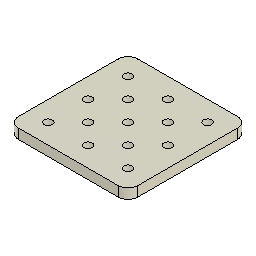
DrillingTool v1 (Autodesk Fusion 360 design; units mm, degrees)
Autodesk Fusion 360 part; units mm, degrees
note: some values were not read from the file. Set by a fixed rule: which sketch regions a step uses.
sketch "Sketch1" plane through (0, 0, 0) normal (0, 0, 1) x (1, 0, 0) in component "inside"
  line L0 (5, 0) -> (55, 0)
  line L1 (60, 5) -> (60, 55)
  line L2 (55, 60) -> (5, 60)
  line L3 (0, 55) -> (0, 5)
  circle A0 centre (10, 10) radius 2.05
  circle A1 centre (30, 10) radius 2.05
  circle A2 centre (10, 30) radius 2.05
  circle A3 centre (30, 30) radius 2.05
  circle A4 centre (50, 10) radius 2.05
  circle A5 centre (50, 30) radius 2.05
  circle A6 centre (20, 40) radius 2.05
  circle A7 centre (40, 40) radius 2.05
  circle A8 centre (10, 50) radius 2.05
  circle A9 centre (30, 50) radius 2.05
  circle A10 centre (50, 50) radius 2.05
  arc A11 (5, 60) -> (0, 55) centre (5, 55) ccw
  arc A12 (60, 55) -> (55, 60) centre (55, 55) ccw
  arc A13 (55, 0) -> (60, 5) centre (55, 5) ccw
  arc A14 (0, 5) -> (5, 0) centre (5, 5) ccw
  circle A15 centre (10, 20) radius 2.05
  circle A16 centre (30, 20) radius 2.05
  circle A17 centre (50, 20) radius 2.05
  circle A18 centre (10, 40) radius 2.05
  circle A19 centre (30, 40) radius 2.05
  circle A20 centre (50, 40) radius 2.05
  circle A21 centre (20, 50) radius 2.05
  circle A22 centre (40, 50) radius 2.05
  circle A23 centre (20, 10) radius 2.05
  circle A24 centre (40, 10) radius 2.05
  circle A25 centre (20, 20) radius 2.05
  circle A26 centre (40, 20) radius 2.05
  circle A27 centre (20, 30) radius 2.05
  circle A28 centre (40, 30) radius 2.05
  dimension "d6" = 60
  dimension "d7" = 60
  dimension "d9" = 4.1
  dimension "d10" = 10
  dimension "d11" = 10
  dimension "d14" = 10
  dimension "d15" = 10
  dimension "d17" = 5
  dimension "d18" = 5
  dimension "d19" = 5
  dimension "d20" = 5
  measures "d9" diameter of A0
  measures "d10" distance of origin
  measures "d11" distance of origin
  measures "d17" radius of A11
  measures "d18" radius of A12
  measures "d19" radius of A13
  measures "d20" radius of A14
extrude "Extrude1" add sketch "Sketch1" along normal blind 5 contours L0 L1 L2 L3 A11 A12 A13 A14 | A15 | A16 | A17 | A18 | A19 | A20 | A21 | A22 | A23 | A24 | A27 | A28 makes body 1 in component "inside"
sketch "Sketch1 (2)" plane through (0, 0, 0) normal (0, 0, 1) x (1, 0, 0) in component "inoutside"
  line L0 (0, -7.5) -> (60, -7.5)
  line L1 (60, -7.5) -> (60, 7.5)
  line L2 (60, 7.5) -> (0, 7.5)
  line L3 (0, 7.5) -> (0, -7.5)
  dimension "d23" = 15
  dimension "d24" = 60
sketch "Sketch2" plane through (0, 0, 0) normal (0, 1, 0) x (1, 0, 0) in component "inoutside"
  line L0 (0, 0) -> (60, 0)
  line L1 (60, 0) -> (60, -55)
  line L2 (55, -60) -> (5, -60)
  line L3 (0, -55) -> (0, 0)
  circle A0 centre (10, -10) radius 2.05
  circle A1 centre (20, -10) radius 2.05
  circle A2 centre (30, -10) radius 2.05
  circle A3 centre (40, -10) radius 2.05
  circle A4 centre (50, -10) radius 2.05
  circle A5 centre (10, -20) radius 2.05
  circle A6 centre (20, -20) radius 2.05
  circle A7 centre (30, -20) radius 2.05
  circle A8 centre (40, -20) radius 2.05
  circle A9 centre (50, -20) radius 2.05
  circle A10 centre (10, -30) radius 2.05
  circle A11 centre (20, -30) radius 2.05
  circle A12 centre (30, -30) radius 2.05
  circle A13 centre (40, -30) radius 2.05
  circle A14 centre (50, -30) radius 2.05
  circle A15 centre (10, -40) radius 2.05
  circle A16 centre (20, -40) radius 2.05
  circle A17 centre (30, -40) radius 2.05
  circle A18 centre (40, -40) radius 2.05
  circle A19 centre (50, -40) radius 2.05
  circle A20 centre (10, -50) radius 2.05
  circle A21 centre (20, -50) radius 2.05
  circle A22 centre (30, -50) radius 2.05
  circle A23 centre (40, -50) radius 2.05
  circle A24 centre (50, -50) radius 2.05
  arc A25 (0, -55) -> (5, -60) centre (5, -55) ccw
  arc A26 (55, -60) -> (60, -55) centre (55, -55) ccw
  dimension "d25" = 60
  dimension "d26" = 60
  dimension "d27" = 4.1
  dimension "d28" = 10
  dimension "d29" = 10
  dimension "d32" = 10
  dimension "d34" = 5
  dimension "d35" = 5
  measures "d27" diameter of A0
  measures "d28" distance of L0.start
  measures "d29" distance of L0.start
  measures "d34" radius of A25
  measures "d35" radius of A26
extrude "Extrude1'" add sketch "Sketch2" along normal mid plane 5 separate body contours L0 L1 L2 L3 A25 A26 | A1 | A3 | A5 | A7 | A9 | A11 | A13 | A15 | A17 | A19 | A21 | A23 makes body 2 in component "inoutside"
extrude "Extrude2" add sketch "Sketch1 (2)" against normal blind 5 bodies 2 in component "inoutside"
sketch "Sketch1 (3)" plane through (0, 0, 0) normal (0, 0, 1) x (1, 0, 0) in component "outside"
  line L0 (0, -7.5) -> (60, -7.5)
  line L1 (60, -7.5) -> (60, 7.5)
  line L2 (60, 7.5) -> (0, 7.5)
  line L3 (0, 7.5) -> (0, -7.5)
  line L4 (0, -7.5) -> (-5, -7.5)
  line L5 (-5, -7.5) -> (-5, 7.5)
  line L6 (-5, 7.5) -> (0, 7.5)
  line L7 (0, 7.5) -> (0, -7.5)
  dimension "d23_1" = 15
  dimension "d24_1" = 60
  dimension "d40" = 5
sketch "Sketch2 (2)" plane through (0, 0, 0) normal (0, 1, 0) x (1, 0, 0) in component "outside"
  line L0 (0, 0) -> (60, 0)
  line L1 (60, 0) -> (60, -55)
  line L2 (55, -60) -> (0, -60)
  line L3 (0, -60) -> (0, 0)
  circle A0 centre (10, -10) radius 2.05
  circle A1 centre (20, -10) radius 2.05
  circle A2 centre (30, -10) radius 2.05
  circle A3 centre (40, -10) radius 2.05
  circle A4 centre (50, -10) radius 2.05
  circle A5 centre (10, -20) radius 2.05
  circle A6 centre (20, -20) radius 2.05
  circle A7 centre (30, -20) radius 2.05
  circle A8 centre (40, -20) radius 2.05
  circle A9 centre (50, -20) radius 2.05
  circle A10 centre (10, -30) radius 2.05
  circle A11 centre (20, -30) radius 2.05
  circle A12 centre (30, -30) radius 2.05
  circle A13 centre (40, -30) radius 2.05
  circle A14 centre (50, -30) radius 2.05
  circle A15 centre (10, -40) radius 2.05
  circle A16 centre (20, -40) radius 2.05
  circle A17 centre (30, -40) radius 2.05
  circle A18 centre (40, -40) radius 2.05
  circle A19 centre (50, -40) radius 2.05
  circle A20 centre (10, -50) radius 2.05
  circle A21 centre (20, -50) radius 2.05
  circle A22 centre (30, -50) radius 2.05
  circle A23 centre (40, -50) radius 2.05
  circle A24 centre (50, -50) radius 2.05
  arc A25 (55, -60) -> (60, -55) centre (55, -55) ccw
  dimension "d25_1" = 60
  dimension "d26_1" = 60
  dimension "d27_1" = 4.1
  dimension "d28_1" = 10
  dimension "d29_1" = 10
  dimension "d32_1" = 10
  dimension "d35_1" = 5
  measures "d27_1" diameter of A0
  measures "d28_1" distance of L0.start
  measures "d29_1" distance of L0.start
  measures "d35_1" radius of A25
extrude "Extrude1''" add sketch "Sketch2 (2)" along normal mid plane 5 separate body contours L0 L1 L2 L3 A25 | A1 | A3 | A5 | A7 | A9 | A11 | A13 | A15 | A17 | A19 | A21 | A23 makes body 3 in component "outside"
extrude "Extrude2'" add sketch "Sketch1 (3)" against normal blind 5 contours L0 L1 L2 L3 L7 bodies 3 in component "outside"
extrude "Extrude3" add sketch "Sketch1 (3)" along normal blind 60 and the other way blind 5 contours L3 L4 L5 L6 L7 bodies 3 in component "outside"
component "inside" placed x (1, 0, 0) y (0, 1, 0) z (0, 0, 1) at (0, 0, 0)
component "inoutside" placed x (1, 0, 0) y (0, 1, 0) z (0, 0, 1) at (0, 0, 0)
component "outside" placed x (1, 0, 0) y (0, 1, 0) z (0, 0, 1) at (0, 0, 0)
equation "length = 60 mm"
equation "thickness = 5 mm"
equation "holesDiameter = 4.1 mm"
equation "holesSpacing = 10 mm"
equation "d6 = length"
equation "d7 = length"
equation "roundingRadius = 5 mm"
equation "d9 = holesDiameter"
equation "d10 = holesSpacing"
equation "d11 = holesSpacing"
equation "d12 = nmbrHoles"
equation "d13 = nmbrHoles"
equation "d14 = holesSpacing"
equation "d15 = holesSpacing"
equation "nmbrHoles = 5"
equation "d17 = roundingRadius"
equation "d18 = roundingRadius"
equation "d19 = roundingRadius"
equation "d20 = roundingRadius"
equation "d21 = thickness"
equation "d23 = 3 * thickness"
equation "d24 = length"
equation "d25 = length"
equation "d26 = length"
equation "d27 = holesDiameter"
equation "d28 = holesSpacing"
equation "d29 = holesSpacing"
equation "d30 = nmbrHoles"
equation "d31 = nmbrHoles"
equation "d32 = holesSpacing"
equation "d33 = -holesSpacing"
equation "d34 = roundingRadius"
equation "d35 = roundingRadius"
equation "d36 = thickness / 2"
equation "d38 = -thickness"
equation "d23_1 = 3 * thickness"
equation "d24_1 = length"
equation "d25_1 = length"
equation "d26_1 = length"
equation "d27_1 = holesDiameter"
equation "d28_1 = holesSpacing"
equation "d29_1 = holesSpacing"
equation "d30_1 = nmbrHoles"
equation "d31_1 = nmbrHoles"
equation "d32_1 = holesSpacing"
equation "d33_1 = -holesSpacing"
equation "d35_1 = roundingRadius"
equation "d36_1 = thickness / 2"
equation "d38_1 = -thickness"
equation "d40 = thickness"
equation "d41 = length"
equation "d43 = thickness"
